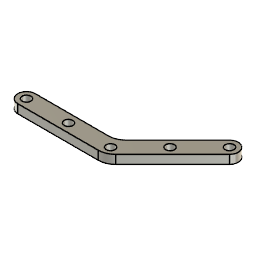
Week1_Bracket (Autodesk Fusion 360 design; units mm, degrees)
part number: 2025-10-11-17-13-09-061
Autodesk Fusion 360 part; units mm, degrees
sketch "Sketch1" plane through (0, 0, 0) normal (0, 0, 1) x (1, 0, 0)
  line L0 (0, 0) -> (458.5786, 0)
  line L1 (529.2893, 29.2893) -> (853.5534, 353.5534)
  line L2 (853.5534, 353.5534) -> (782.8427, 424.2641) construction
  line L3 (782.8427, 424.2641) -> (487.868, 129.2893)
  line L4 (417.1573, 100) -> (0, 100)
  line L5 (0, 100) -> (0, 0) construction
  circle A0 centre (818.1981, 388.9087) radius 50
  circle A1 centre (0, 50) radius 50
  arc A2 (417.1573, 100) -> (487.868, 129.2893) centre (417.1573, 200) ccw
  arc A3 (458.5786, 0) -> (529.2893, 29.2893) centre (458.5786, 100) ccw
  dimension "d1" = 45
  dimension "d2" = 100
  dimension "d3" = 100
  dimension "d4" = 100
  dimension "d5" = 100
  constraint coincident L0.start L5.end
  constraint horizontal L0
  constraint perpendicular L1 L2
  constraint perpendicular L2 L3
  constraint horizontal L4
  constraint perpendicular L0 L5
  constraint equal L2 L5
  constraint midpoint L2 A0.centre
  constraint midpoint L5 A1.centre
  constraint tangent L3 A2
  constraint tangent L4 A2
  constraint tangent L0 A3
  constraint tangent L1 A3
  constraint equal A2 A3
  measures "d1" angle of L0 L1
  measures "d2" distance of L1.end L2.end
  measures "d3" diameter of A0
  measures "d4" diameter of A1
  measures "d5" radius of A2
extrude "Extrude1" add sketch "Sketch1" along normal blind 50
sketch "Sketch2" plane through (0, 0, 50) normal (0, 0, 1) x (-1, 0, 0)
  line L0 (-417.1573, -100) -> (0, -100)
  arc A0 (0, -100) -> (0, 0) centre (0, -50) ccw
  line L1 (0, 0) -> (-458.5786, 0)
  arc A1 (-458.5786, 0) -> (-529.2893, -29.2893) centre (-458.5786, -100) ccw
  line L2 (-529.2893, -29.2893) -> (-853.5534, -353.5534)
  arc A2 (-853.5534, -353.5534) -> (-782.8427, -424.2641) centre (-818.1981, -388.9087) ccw
  line L3 (-782.8427, -424.2641) -> (-487.868, -129.2893)
  arc A3 (-417.1573, -100) -> (-487.868, -129.2893) centre (-417.1573, -200) ccw
  line L4 (0, -50) -> (-479.2893, -50) construction
  line L5 (-479.2893, -50) -> (-818.1981, -388.9087) construction
  circle A4 centre (0, -50) radius 25
  circle A5 centre (-239.6447, -50) radius 25
  circle A6 centre (-479.2893, -50) radius 25
  circle A7 centre (-648.7437, -219.4544) radius 25
  circle A8 centre (-818.1981, -388.9087) radius 25
  dimension "d8" = 50
  dimension "d9" = 50
  dimension "d10" = 50
  dimension "d11" = 50
  dimension "d12" = 50
  constraint coincident A0.centre L4.start
  constraint parallel L1 L4
  constraint coincident A2.centre L5.end
  constraint parallel L2 L5
  constraint midpoint L4 A5.centre
  constraint coincident L4.end L5.start
  constraint midpoint L5 A7.centre
  measures "d8" diameter of A4
  measures "d9" diameter of A5
  measures "d10" diameter of A6
  measures "d11" diameter of A7
  measures "d12" diameter of A8
extrude "Extrude2" cut sketch "Sketch2" against normal blind 200 contours A4 | A5 | A6 | A7 | A8
